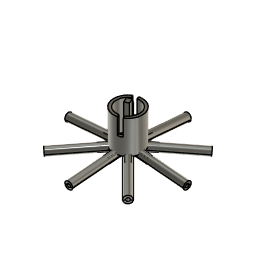
turnstileSupport5deg (Autodesk Fusion 360 design; units mm, degrees)
Autodesk Fusion 360 part; units mm, degrees
cylinder "CylinderPrimitive1" add diameter 52 height 60 placed x (1, 0, 0) y (0, 1, 0) z (0, 0, 1) at (0, 0, 0) makes body 1
hole "Hole1" at (0, 0, 60) direction (0, 0, -1) diameter 42.2 depth 55 tip angle 180 bodies 1
hole "Hole2" at (0, 0, 0) direction (0, 0, 1) diameter 33.75 depth 55 tip angle 180 bodies 1
cylinder "CylinderPrimitive2" add diameter 14 height 90 placed x (1, 0, 0) y (0, 0, -1) z (0, 1, 0) at (0, 0, 0) separate body makes body 2
move_body "Move1" bodies 2 to x (1, 0, 0) y (0, 1, 0) z (0, 0, 1) at (0, 15, 2)
move_body "Move2" bodies 2 to x (1, 0, 0) y (0, 1, 0) z (0, 0, 1) at (0, 2, -1)
box "BoxPrimitive1" add length 22 width 8 height -10 placed x (0, -1, 0) y (1, 0, 0) z (0, 0, 1) at (-3, 10, 0) separate body makes body 3
move_body "Move3" bodies 3 to x (1, 0, 0) y (0, 1, 0) z (0, 0, 1) at (-1, 29, 6)
extrude "Extrude1" cut 1 faces at (-1.3333, 17, -0.6667) along direction (0, 1, 0) blind 22 on bodies 3 bodies 1 2 3
move_body "Move36" bodies 2 to x (1, 0, 0) y (0, 0.996195, -0.087156) z (0, 0.087156, 0.996195) at (0, 0.0194, -14.5558)
extrude "Extrude55" add 1 faces at (1.3333, 17, 1.6667) along direction (0, 1, 0) blind 6 on bodies 1 bodies 1 3
extrude "Extrude56" add 1 faces at (-3.1135, 22.4884, 6) along direction (0, 0, -1) blind 6 on bodies 1 bodies 1
hole "Hole10" at (0, 106.6994, -22.8853) direction (0, -0.996195, 0.087156) diameter 6.3 depth 90 tip angle 180 bodies 2
move_body "Move37" bodies 2 to x (1, 0, 0) y (0, 1, 0) z (0, 0, 1) at (0, 1.133, 12.9505)
extrude "Extrude57" cut 1 faces at (0, 39.7091, -8.3748) along direction (0, -0.996195, 0.087156) blind 22 on bodies 2 bodies 1
extrude "Extrude58" cut 1 faces at (-1.3333, 25.9161, 2.2511) along direction (0, -0.087156, -0.996195) blind 6 on bodies 2 bodies 1
move_body "Move38" bodies 2 to x (1, 0, 0) y (0, 1, 0) z (0, 0, 1) at (0, 0, -17)
move_body "Move39" bodies 2 to x (1, 0, 0) y (0, 0.996195, 0.087156) z (0, -0.087156, 0.996195) at (0, -2.8884, -1.6599)
split "Split6" by plane through (0, 0, -20) normal (0, 0, 1) bodies 2 makes body 4 at (6.9914, 76.8811, -18.7471)
move_body "Move40" bodies 4 2 to x (1, 0, 0) y (0, 0.996195, -0.087156) z (0, 0.087156, 0.996195) at (0, 1.5918, 2.3651)
move_body "Move41" bodies 4 2 to x (1, 0, 0) y (0, 1, 0) z (0, 0, 1) at (0, 1.3945, 15.9391)
copy_body "CopyPasteBodies14" bodies 2 4 makes body 5 makes body 6
move_body "Move42" bodies 5 6 to x (-1, 0, 0) y (0, -1, 0) z (0, 0, 1) at (0, 0, 0)
copy_body "CopyPasteBodies15" bodies 2 4 6 5 makes body 7 makes body 8 makes body 9 makes body 10
move_body "Move43" bodies 7 8 9 10 to x (0, -1, 0) y (1, 0, 0) z (0, 0, 1) at (0, 0, 0)
copy_body "CopyPasteBodies16" bodies 4 2 8 7 6 5 10 9 makes body 11 makes body 12 makes body 13 makes body 14 makes body 15 makes body 16 makes body 17 makes body 18
move_body "Move44" bodies 11 12 13 14 15 16 17 18 to x (0.707107, -0.707107, 0) y (0.707107, 0.707107, 0) z (0, 0, 1) at (0, 0, 0)
box "BoxPrimitive7" add length 10 width 8 height 40 placed x (0, 1, 0) y (-1, 0, 0) z (0, 0, 1) at (5, -3, 0) separate body makes body 19
move_body "Move45" bodies 19 to x (1, 0, 0) y (0, 1, 0) z (0, 0, 1) at (0, 0, 30)
move_body "Move46" bodies 19 to x (1, 0, 0) y (0, 1, 0) z (0, 0, 1) at (-1, -2, 0)
move_body "Move47" bodies 19 to x (0.92388, 0.382683, 0) y (-0.382683, 0.92388, 0) z (0, 0, 1) at (0, 0, 0)
extrude "Extrude59" cut 1 faces at (0.6816, -5.1296, 43.3333) along direction (0.382683, -0.92388, 0) blind 33 on bodies 19 bodies 1
extrude "Extrude60" cut 1 faces at (-3.1453, 4.1092, 43.3333) along direction (-0.382683, 0.92388, 0) blind 45 on bodies 19 bodies 1
extrude "Extrude61" cut 1 faces at (25.8803, 1.3333, 2.1535) along direction (-0.087156, 0, -0.996195) blind 3 on bodies 8 bodies 1
extrude "Extrude62" cut 1 faces at (19.2429, 17.3573, 2.1535) along direction (-0.061628, -0.061628, -0.996195) blind 4 on bodies 11 bodies 1
extrude "Extrude63" cut 1 faces at (-22.523, 24.4087, 1.5143) along direction (0.061628, -0.061628, -0.996195) blind 4 on bodies 18 bodies 1
extrude "Extrude64" cut 1 faces at (-33.1857, -1.3333, 1.5143) along direction (0.087156, 0, -0.996195) blind 5 on bodies 9 bodies 1
extrude "Extrude65" cut 1 faces at (-19.2429, -17.3573, 2.1535) along direction (0.061628, 0.061628, -0.996195) blind 5 on bodies 15 bodies 1
extrude "Extrude66" cut 1 faces at (1.3333, -25.8803, 2.1535) along direction (0, 0.087156, -0.996195) blind 4 on bodies 6 bodies 1
extrude "Extrude67" cut 1 faces at (22.523, -24.4087, 1.5143) along direction (-0.061628, 0.061628, -0.996195) blind 5 on bodies 13 bodies 1
hole "Hole3" [rolled back] hole depth 95 hole diameter 6.2 tip angle 180
split "Split1" [rolled back]
extrude "Extrude2" [rolled back] along distance -105 taper angle 0
extrude "Extrude3" [rolled back] along distance -4 taper angle 0
split "Split2" [rolled back]
move_body "Move4" [rolled back]
extrude "Extrude4" [rolled back] along distance -5 taper angle 0
move_body "Move5" [rolled back]
combine "Combine1" [rolled back]
pasted_body "CopyPasteBodies1" makes body 20
move_body "Move6" [rolled back]
pasted_body "CopyPasteBodies2" makes body 21 makes body 22
move_body "Move7" [rolled back]
extrude "Extrude5" [rolled back] along distance 69 taper angle 0
extrude "Extrude6" [rolled back] along distance 31 taper angle 0
extrude "Extrude7" [rolled back] along distance -4.5 taper angle 0
extrude "Extrude8" [rolled back] along distance -0.5 taper angle 0
extrude "Extrude9" [rolled back] along distance -0.5 taper angle 0
extrude "Extrude10" [rolled back] along distance -0.1 taper angle 0
extrude "Extrude11" [rolled back] along distance -0.1 taper angle 0
hole "Hole4" [rolled back] hole depth 20 hole diameter 7.5 tip angle 180
hole "Hole5" [rolled back] hole depth 20 hole diameter 7.5 tip angle 180
cylinderprimitive "CylinderPrimitive3" [rolled back] height 90 diameter 14
move_body "Move8" [rolled back]
hole "Hole6" [rolled back] hole depth 95 hole diameter 3.3 tip angle 180
boxprimitive "BoxPrimitive2" [rolled back] distance x 8 distance y 22 distance z -10 offset distance x 0 offset distance y 0
move_body "Move9" [rolled back]
extrude "Extrude12" [rolled back] along distance -22 taper angle 0
extrude "Extrude13" [rolled back] along distance 36 taper angle 0
split "Split3" [rolled back]
extrude "Extrude14" [rolled back] along distance -101 taper angle 0
moveface "MoveFace1" [rolled back]
extrude "Extrude15" [rolled back] along distance 26 taper angle 0
hole "Hole7" [rolled back] hole depth 20 hole diameter 6 tip angle 180
extrude "Extrude16" [rolled back] along distance 36 taper angle 0
hole "Hole8" [rolled back] hole depth 20 hole diameter 6 tip angle 180
extrude "Extrude17" [rolled back] along distance 30 taper angle 0
hole "Hole9" [rolled back] hole depth 20 hole diameter 6 tip angle 180
extrude "Extrude18" [rolled back] along distance 10 taper angle 0
extrude "Extrude19" [rolled back] along distance 30 taper angle 0
extrude "Extrude20" [rolled back] along distance 110 taper angle 0
extrude "Extrude21" [rolled back] along distance 205 taper angle 0
boxprimitive "BoxPrimitive3" [rolled back] distance x 15 distance y 15 distance z 45 offset distance x 0 offset distance y 0
fillet "Fillet1" [rolled back] radius 2.5
move_body "Move16" [rolled back]
move_body "Move17" [rolled back]
move_body "Move18" [rolled back]
pasted_body "CopyPasteBodies5" makes body 23
move_body "Move19" [rolled back]
combine "Combine2" [rolled back]
fillet "Fillet2" [rolled back] radius 3
fillet "Fillet3" [rolled back] radius 3
boxprimitive "BoxPrimitive4" [rolled back] distance x 51 distance y 4 distance z 2 offset distance x 0 offset distance y 0
extrude "Extrude22" [rolled back] along distance 44 taper angle 0
move_body "Move20" [rolled back]
move_body "Move21" [rolled back]
extrude "Extrude23" [rolled back] along distance 26 taper angle 0
combine "Combine3" [rolled back]
pasted_body "CopyPasteBodies6" makes body 24
move_body "Move22" [rolled back]
pasted_body "CopyPasteBodies7" makes body 25 makes body 26
move_body "Move23" [rolled back]
pasted_body "CopyPasteBodies8" makes body 27 makes body 28 makes body 29 makes body 30
move_body "Move24" [rolled back]
delete_body "RemoveBody1" bodies 31
pasted_body "CopyPasteBodies9" makes body 32 makes body 33 makes body 34 makes body 35
move_body "Move25" [rolled back]
split "Split4" [rolled back]
delete_body "RemoveBody2" bodies 36
extrude "Extrude24" [rolled back] along distance 100 taper angle 0
boxprimitive "BoxPrimitive5" [rolled back] distance x 15 distance y 10 distance z 70 offset distance x 0 offset distance y 0
move_body "Move26" [rolled back]
move_body "Move27" [rolled back]
move_body "Move28" [rolled back]
pasted_body "CopyPasteBodies10" makes body 37
move_body "Move29" [rolled back]
extrude "Extrude25" [rolled back] along distance -100 taper angle 0
split "Split5" [rolled back]
delete_body "RemoveBody3" bodies 38
extrude "Extrude26" [rolled back] along distance 100 taper angle 0
extrude "Extrude27" [rolled back] along distance -20 taper angle 0
extrude "Extrude28" [rolled back] along distance -40 taper angle 0
fillet "Fillet4" [rolled back] radius 8
fillet "Fillet5" [rolled back] radius 8
fillet "Fillet6" [rolled back] radius 8
fillet "Fillet7" [rolled back] radius 8
extrude "Extrude29" [rolled back] along distance -10 taper angle 0
extrude "Extrude30" [rolled back] along distance -10 taper angle 0
fillet "Fillet8" [rolled back] radius 5
fillet "Fillet9" [rolled back] radius 5
extrude "Extrude31" [rolled back] along distance 1 taper angle 0
extrude "Extrude32" [rolled back] along distance 1 taper angle 0
boxprimitive "BoxPrimitive6" [rolled back] distance x 4 distance y 4 distance z 25 offset distance x 0 offset distance y 0
move_body "Move30" [rolled back]
move_body "Move31" [rolled back]
extrude "Extrude33" [rolled back] along distance 1 taper angle 0
extrude "Extrude34" [rolled back] along distance 1 taper angle 0
move_body "Move32" [rolled back]
pasted_body "CopyPasteBodies11" makes body 39
move_body "Move33" [rolled back]
pasted_body "CopyPasteBodies12" makes body 40 makes body 41
move_body "Move34" [rolled back]
pasted_body "CopyPasteBodies13" makes body 42 makes body 43 makes body 44 makes body 45
move_body "Move35" [rolled back]
extrude "Extrude35" [rolled back] along distance 1 taper angle 0
extrude "Extrude36" [rolled back] along distance 1 taper angle 0
extrude "Extrude37" [rolled back] along distance 1 taper angle 0
extrude "Extrude38" [rolled back] along distance 1 taper angle 0
extrude "Extrude39" [rolled back] along distance 1 taper angle 0
extrude "Extrude40" [rolled back] along distance 1 taper angle 0
extrude "Extrude41" [rolled back] along distance 1 taper angle 0
extrude "Extrude42" [rolled back] along distance 1 taper angle 0
extrude "Extrude43" [rolled back] along distance 1 taper angle 0
extrude "Extrude44" [rolled back] along distance 1 taper angle 0
extrude "Extrude45" [rolled back] along distance 1 taper angle 0
extrude "Extrude46" [rolled back] along distance 1 taper angle 0
extrude "Extrude47" [rolled back] along distance 22 taper angle 0
extrude "Extrude48" [rolled back] along distance 22 taper angle 0
extrude "Extrude49" [rolled back] along distance 22 taper angle 0
extrude "Extrude50" [rolled back] along distance 22 taper angle 0
extrude "Extrude51" [rolled back] along distance 22 taper angle 0
extrude "Extrude52" [rolled back] along distance 22 taper angle 0
extrude "Extrude53" [rolled back] along distance 22 taper angle 0
extrude "Extrude54" [rolled back] along distance 23 taper angle 0
combine "Combine5" [rolled back]
combine "Combine4" [suppressed]
